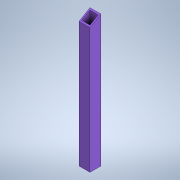
# Autodesk Inventor part: sideAluminumExtrusion
Saved by Autodesk Inventor 2020.2 (Build 242310000, 310)
## iProperties
Created: 2020-01-19
Part Number: sideAluminumExtrusion
Material: Aluminum 6061, Welded
Document SubType Name: Modeling
Designer: robst
Density: 2.7 g/cm^3
Appearance: Violet
Author: robst
Autodesk Inventor part; units mm, degrees
ref_plane "YZ Plane" through (0, 0, 0) normal (1, 0, 0) x (0, 1, 0)
ref_plane "XZ Plane" through (0, 0, 0) normal (0, 1, 0) x (-1, 0, 0)
ref_plane "XY Plane" through (0, 0, 0) normal (0, 0, 1) x (1, 0, 0)
sketch "Sketch1" plane through (0, 0, 0) normal (0, 1, 0) x (-1, 0, 0)
  line L0 (12.7, 12.7) -> (-12.7, 12.7)
  line L1 (-12.7, 12.7) -> (-12.7, -12.7)
  line L2 (-12.7, -12.7) -> (12.7, -12.7)
  line L3 (12.7, -12.7) -> (12.7, 12.7)
  line L4 (12.7, 12.7) -> (-12.7, -12.7) construction
  line L5 (-12.7, 12.7) -> (12.7, -12.7) construction
  line L6 (9.525, 9.525) -> (-9.525, 9.525)
  line L7 (-9.525, 9.525) -> (-9.525, -9.525)
  line L8 (-9.525, -9.525) -> (9.525, -9.525)
  line L9 (9.525, -9.525) -> (9.525, 9.525)
  line L10 (9.525, 9.525) -> (-9.525, -9.525) construction
  line L11 (-9.525, 9.525) -> (9.525, -9.525) construction
  point P0 (0, 0)
  dimension "d0" = 25.4
  dimension "d1" = 25.4
  dimension "d2" = 3.175
  constraints: 24 end point, 4 midpoint, 4 parallel, 3 perpendicular, 2 horizontal
  measures "d0" distance of L0.start L0.end
  measures "d1" distance of L1.end L0.end
  measures "d2" distance between parallel lines of L6 L0
extrude "Extrusion1" add sketch "Sketch1" along normal mid plane 304.8
sketch "Sketch2" plane through (12.7, -152.4, -12.7) normal (1, 0, 0) x (0, 0, -1)
  line L0 (0, 0) -> (0, 304.8) projected
  line L1 (0, 304.8) -> (-25.4, 290.1353)
  line L2 (-25.4, 0) -> (-25.4, 304.8) projected
  line L3 (-25.4, 304.8) -> (0, 304.8)
  point P0 (-12.7, 152.4)
  dimension "d8" = 30
  constraints: 4 end point, 1 perpendicular, 1 point on line
  measures "d8" angle of L3 L1
extrude "Extrusion2" cut sketch "Sketch2" against normal through all
body "Solid1"
